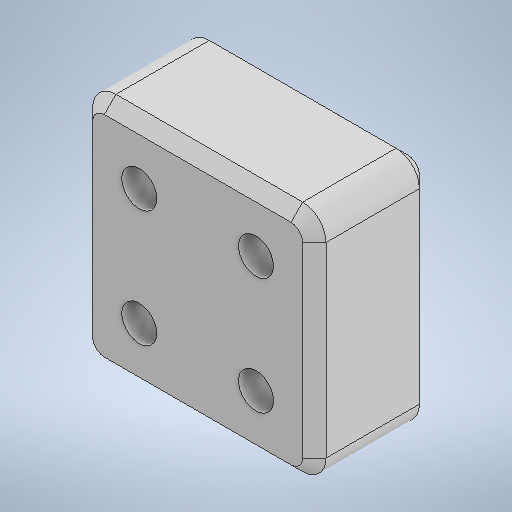
# Autodesk Inventor part: RobotBaseConnector
Saved by Autodesk Inventor 2025.3 (Build 293356000, 356)
## iProperties
Created: 2025-04-28
Part Number: RobotBaseConnector
Material: 일반
Document SubType Name: Modeling
Designer: SEON
Density: 1 g/cm^3
Appearance: 기본값
Author: SEON
## iProperties of the stored document RobotBaseConnector_3D 인쇄.ipt
Created: 2025-05-11
Part Number: RobotBaseConnector_3D 인쇄
Material: 일반
Document SubType Name: Modeling
Designer: SEON
Density: 1 g/cm^3
Appearance: 기본값
Author: SEON
Autodesk Inventor part; units mm, degrees
ref_plane "YZ Plane" through (0, 0, 0) normal (1, 0, 0) x (0, 1, 0)
ref_plane "XZ Plane" through (0, 0, 0) normal (0, 1, 0) x (-1, 0, 0)
ref_plane "XY Plane" through (0, 0, 0) normal (0, 0, 1) x (1, 0, 0)
sketch "스케치1" plane through (0, 0, 0) normal (0, 0, 1) x (1, 0, 0)
  line L0 (-10, -10) -> (10, -10)
  line L1 (10, -10) -> (10, 10)
  line L2 (10, 10) -> (-10, 10)
  line L3 (-10, 10) -> (-10, -10)
  line L4 (-10, -10) -> (10, 10) construction
  line L5 (10, -10) -> (-10, 10) construction
  circle A0 centre (-5, 5) radius 1.5
  circle A1 centre (5, 5) radius 1.5
  circle A2 centre (5, -5) radius 1.5
  circle A3 centre (-5, -5) radius 1.5
  point P0 (0, 0)
  dimension "d0" = 20
  dimension "d1" = 5
  dimension "d2" = 3
  constraints: 12 end point, 4 centre point, 4 point on line, 3 equal radius, 2 horizontal alignment, 2 midpoint, 2 parallel, 2 perpendicular, 2 vertical alignment, 1 horizontal
  measures "d0" distance of L0.end L1.end
  measures "d1" distance from line of L2 A1.centre
  measures "d2" diameter of A0
extrude "돌출1" add sketch "스케치1" along normal blind 10
fillet "모깎기1" radius 2 4 edges at (-10, 10, 5) (-10, -10, 5) (10, -10, 5) (10, 10, 5)
chamfer "모따기1" distance 1 angle 45 16 edges at (0, 10, 10) (-9.4142, 9.4142, 10) (-10, 0, 10) (-9.4142, -9.4142, 10) (0, -10, 10) (9.4142, -9.4142, 10) (10, 0, 10) (9.4142, 9.4142, 10) (0, 10, 0) (-9.4142, 9.4142, 0) (-10, 0, 0) (-9.4142, -9.4142, 0) (0, -10, 0) (9.4142, -9.4142, 0) (10, 0, 0) (9.4142, 9.4142, 0)
